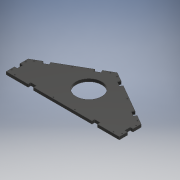
# Autodesk Inventor part: BA01
Saved by Autodesk Inventor 2017 (Build 210142000, 142)
## iProperties
Created: 2019-05-22
Part Number: BA01
Material: Polyethylene, High Density
Document SubType Name: Modeling
Designer: Dell
Density: 0.952 g/cm^3
Appearance: Smooth - Black
Author: Dell
Autodesk Inventor part; units mm, degrees
ref_plane "YZ Plane" through (0, 0, 0) normal (1, 0, 0) x (0, 1, 0)
ref_plane "XZ Plane" through (0, 0, 0) normal (0, 1, 0) x (-1, 0, 0)
ref_plane "XY Plane" through (0, 0, 0) normal (0, 0, 1) x (1, 0, 0)
sketch "Sketch1" plane through (0, 0, 0) normal (0, 0, 1) x (1, 0, 0)
  line L0 (0, 0) -> (0, 101.6)
  line L1 (0, 0) -> (525.78, 0)
  line L2 (525.78, 0) -> (525.78, 101.6)
  line L3 (525.78, 101.6) -> (262.89, 253.3796)
  line L4 (262.89, 253.3796) -> (0, 101.6)
  circle A0 centre (262.89, 121.3796) radius 60
  line L5 (6.35, 97.9338) -> (6.35, 6.35) construction
  line L6 (6.35, 6.35) -> (519.43, 6.35) construction
  line L7 (519.43, 6.35) -> (519.43, 97.9338) construction
  line L8 (519.43, 97.9338) -> (262.89, 246.0473) construction
  line L9 (262.89, 246.0473) -> (6.35, 97.9338) construction
  line L10 (12.7, 94.2677) -> (12.7, 12.7) construction
  line L11 (12.7, 12.7) -> (513.08, 12.7) construction
  line L12 (513.08, 12.7) -> (513.08, 94.2677) construction
  line L13 (513.08, 94.2677) -> (262.89, 238.7149) construction
  line L14 (262.89, 238.7149) -> (12.7, 94.2677) construction
  circle A1 centre (6.35, 84.6419) radius 2.25
  circle A2 centre (6.35, 19.6419) radius 2.25
  line L15 (6.35, 84.6419) -> (6.35, 19.6419) construction
  circle A3 centre (32.89, 6.35) radius 2.25
  circle A4 centre (212.89, 6.35) radius 2.25
  circle A5 centre (312.89, 6.35) radius 2.25
  circle A6 centre (492.89, 6.35) radius 2.25
  line L16 (32.89, 6.35) -> (492.89, 6.35) construction
  line L17 (212.89, 6.35) -> (312.89, 6.35) construction
  line L18 (22.0367, 106.9905) -> (247.2033, 236.9905) construction
  circle A7 centre (22.0367, 106.9905) radius 2.25
  circle A8 centre (247.2033, 236.9905) radius 2.25
  line L19 (262.89, 0) -> (262.89, 253.3796) construction
  circle A9 centre (519.43, 84.6419) radius 2.25
  circle A10 centre (519.43, 19.6419) radius 2.25
  circle A11 centre (503.7433, 106.9905) radius 2.25
  circle A12 centre (278.5767, 236.9905) radius 2.25
  circle A13 centre (134.62, 171.9905) radius 2.25
  circle A14 centre (391.16, 171.9905) radius 2.25
  point P0 (6.35, 52.1419)
  point P1 (6.35, 52.1419)
  point P2 (262.89, 6.35)
  point P3 (262.89, 6.35)
  point P4 (262.89, 6.35)
  dimension "d0" = 101.6
  dimension "d1" = 525.78
  dimension "d2" = 120
  dimension "d3" = 120
  dimension "d4" = 121.3796
  dimension "d5" = 6.35
  dimension "d6" = 6.35
  dimension "d7" = 4.5
  dimension "d8" = 4.5
  dimension "d9" = 65
  dimension "d10" = 4.5
  dimension "d11" = 4.5
  dimension "d12" = 4.5
  dimension "d13" = 4.5
  dimension "d14" = 460
  dimension "d15" = 100
  dimension "d16" = 4.5
  dimension "d17" = 4.5
  dimension "d18" = 260
  dimension "d33" = 4.5
  dimension "d34" = 4.5
  constraints: 40 end point, 15 centre point, 9 midpoint, 8 point on line, 6 coincident, 4 perpendicular, 4 symmetric about line, 2 collinear, 2 vertical alignment, 1 horizontal, 1 horizontal alignment, 1 parallel, 1 vertical, 12 other
  measures "d0" distance of L0.start L0.end
  measures "d1" distance of L0.start L1.end
  measures "d2" angle of L0 L4
  measures "d3" diameter of A0
  measures "d4" distance of L19.start A0.centre
  measures "d5" distance between parallel lines of L4 L9
  measures "d6" distance between parallel lines of L9 L14
  measures "d7" diameter of A1
  measures "d8" diameter of A2
  measures "d9" distance of L15.end L15.start
  measures "d10" diameter of A3
  measures "d11" diameter of A4
  measures "d12" diameter of A5
  measures "d13" diameter of A6
  measures "d14" distance of L16.end L16.start
  measures "d15" distance of L17.end L17.start
  measures "d16" diameter of A7
  measures "d17" diameter of A8
  measures "d18" distance of L18.end L18.start
  measures "d33" diameter of A13
  measures "d34" diameter of A14
extrude "Extrusion1" add sketch "Sketch1" along normal blind 12.7
sketch "Sketch2" plane through (0, 0, 0) normal (0, 0, -1) x (-1, 0, 0)
  line L0 (-101.6, 12.7) -> (-127, 12.7)
  line L1 (-127, 12.7) -> (-127, 0)
  line L2 (-127, 0) -> (-101.6, 0)
  line L3 (-101.6, 0) -> (-101.6, 12.7)
  line L4 (-525.78, 0) -> (0, 0) projected
  line L5 (0, 0) -> (0, 101.6) projected
  line L6 (0, 0) -> (-525.78, 0) projected
  line L7 (-262.89, 0) -> (-262.89, -49.0023)
  line L8 (-424.18, 12.7) -> (-398.78, 12.7)
  line L9 (-398.78, 12.7) -> (-398.78, 0)
  line L10 (-398.78, 0) -> (-424.18, 0)
  line L11 (-424.18, 0) -> (-424.18, 12.7)
  line L12 (0, 0) -> (-525.78, 0)
  line L13 (-525.78, 0) -> (0, 0)
  line L14 (0, 101.6) -> (0, 0) projected
  line L15 (0, 38.1) -> (-12.7, 38.1)
  line L16 (-12.7, 38.1) -> (-12.7, 63.5)
  line L17 (-12.7, 63.5) -> (0, 63.5)
  line L18 (0, 63.5) -> (0, 38.1)
  line L19 (-525.78, 0) -> (-525.78, 101.6)
  line L20 (-525.78, 101.6) -> (-525.78, 0)
  line L21 (-525.78, 38.1) -> (-513.08, 38.1)
  line L22 (-513.08, 38.1) -> (-513.08, 63.5)
  line L23 (-513.08, 63.5) -> (-525.78, 63.5)
  line L24 (-525.78, 63.5) -> (-525.78, 38.1)
  point P0 (0, 50.8)
  point P1 (-525.78, 50.8)
  dimension "d21" = 25.4
  dimension "d22" = 12.7
  dimension "d23" = 101.6
  dimension "d26" = 12.7
  dimension "d27" = 25.4
  constraints: 42 end point, 13 symmetric about line, 4 parallel, 4 point on line, 3 midpoint, 2 horizontal, 2 perpendicular, 1 vertical
  measures "d21" distance of L2.end L1.end
  measures "d22" distance of L1.end L0.end
  measures "d23" distance between parallel lines of L5 L3
  measures "d26" distance of L16.end L17.end
  measures "d27" distance of L15.end L16.end
extrude "Extrusion2" cut sketch "Sketch2" against normal through all
sketch "Sketch3" plane through (0, 0, 0) normal (0, 0, -1) x (-1, 0, 0)
  line L0 (0, 101.6) -> (-262.89, 253.3796) projected
  line L1 (-43.9941, 127) -> (-50.3441, 116.0015)
  line L2 (-50.3441, 116.0015) -> (-72.3411, 128.7015)
  line L3 (-72.3411, 128.7015) -> (-65.9911, 139.7)
  line L4 (-65.9911, 139.7) -> (-43.9941, 127)
  line L5 (-131.445, 177.4898) -> (-144.4004, 155.0504)
  line L6 (-262.89, 253.3796) -> (0, 101.6)
  line L7 (-218.8959, 227.9796) -> (-225.2459, 216.9811)
  line L8 (-225.2459, 216.9811) -> (-203.2489, 204.2811)
  line L9 (-203.2489, 204.2811) -> (-196.8989, 215.2796)
  line L10 (-196.8989, 215.2796) -> (-218.8959, 227.9796)
  point P0 (0, 0)
  dimension "d28" = 12.7
  dimension "d29" = 25.4
  dimension "d30" = 50.8
  constraints: 20 end point, 6 symmetric about line, 3 perpendicular, 2 parallel, 2 point on line, 1 midpoint
  measures "d28" distance of L1.start L1.end
  measures "d29" distance of L1.end L2.end
  measures "d30" distance from line of L0.start L1
extrude "Extrusion3" cut sketch "Sketch3" against normal through all
ref_plane "Work Plane1" through (262.89, 0, 0) normal (-1, 0, 0) x (0, 0, 1)
mirror "Mirror1" about plane through (262.89, 0, 0) normal (-1, 0, 0) of "Extrusion3"
body "Solid1"
